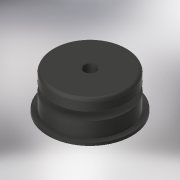
# Autodesk Inventor part: Bauteil1
Saved by Autodesk Inventor 2018 (Build 220112000, 112)
## iProperties
Part Number: Bauteil1
Material: Generisch
Document SubType Name: Modeling
Designer: fufablab07
Density: 1 g/cm^3
Appearance: Glatt - schwarz
Author: fufablab07
Autodesk Inventor part; units mm, degrees
ref_plane "YZ Plane" through (0, 0, 0) normal (1, 0, 0) x (0, 1, 0)
ref_plane "XZ Plane" through (0, 0, 0) normal (0, 1, 0) x (-1, 0, 0)
ref_plane "XY Plane" through (0, 0, 0) normal (0, 0, 1) x (1, 0, 0)
sketch "Skizze1" plane through (0, 0, 0) normal (0, 0, 1) x (1, 0, 0)
  circle A0 centre (0, 0) radius 22.035
  dimension "d0" = 44.07
  constraints: 1 centre point, 1 coincident
  measures "d0" diameter of A0
extrude "Extrusion1" add sketch "Skizze1" along normal blind 1.5
sketch "Skizze2" plane through (0, 0, 1.5) normal (0, 0, 1) x (1, 0, 0)
  circle A0 centre (0, 0) radius 19.5
  dimension "d3" = 39
  constraints: 1 centre point, 1 coincident
  measures "d3" diameter of A0
extrude "Extrusion2" add sketch "Skizze2" along normal blind 8
sketch "Skizze3" plane through (0, 0, 9.5) normal (0, 0, 1) x (1, 0, 0)
  circle A0 centre (0, 0) radius 9.75
  dimension "d6" = 19.5
  constraints: 1 centre point, 1 coincident
  measures "d6" diameter of A0
extrude "Extrusion3" add sketch "Skizze3" along normal blind 4.2
sketch "Skizze4" plane through (0, 0, 13.7) normal (0, 0, 1) x (1, 0, 0)
  circle A0 centre (0, 0) radius 19.5
  dimension "d12" = 39
  constraints: 1 centre point, 1 coincident
  measures "d12" diameter of A0
extrude "Extrusion4" add sketch "Skizze4" along normal blind 6
fillet "Rundung1" radius 1.5 1 edges at (-19.5, 0, 19.7)
sketch "Skizze5" plane through (0, 0, 19.7) normal (0, 0, 1) x (1, 0, 0)
  circle A0 centre (0, 0) radius 3.25
  dimension "d13" = 6.5
  constraints: 1 centre point, 1 coincident
  measures "d13" diameter of A0
extrude "Extrusion5" cut sketch "Skizze5" against normal blind 100
